Autodesk Inventor part; units mm, degrees
(part 2 of 2)
sketch "Sketch10" plane through (0, 6.35, 0) normal (0, 1, 0) x (1, 0, 0)
  line L0 (-0.1825, 29.2815) -> (-0.1825, 141.0415) projected
  arc A0 (-2.7225, 26.7415) -> (-0.1825, 29.2815) centre (-2.7225, 29.2815) ccw projected
  line L1 (-50.9825, 26.7415) -> (-2.7225, 26.7415) projected
  arc A1 (-53.5225, 29.2815) -> (-50.9825, 26.7415) centre (-50.9825, 29.2815) ccw projected
  line L2 (-53.5225, 141.0415) -> (-53.5225, 29.2815) projected
  arc A2 (-50.9825, 143.5815) -> (-53.5225, 141.0415) centre (-50.9825, 141.0415) ccw projected
  line L3 (-2.7225, 143.5815) -> (-50.9825, 143.5815) projected
  arc A3 (-0.1825, 141.0415) -> (-2.7225, 143.5815) centre (-2.7225, 141.0415) ccw projected
  line L4 (-2.405, 141.994) -> (-2.405, 141.359) projected
  line L5 (-3.04, 141.994) -> (-2.405, 141.994) projected
  line L6 (-3.04, 141.359) -> (-3.04, 141.994) projected
  line L7 (-2.405, 141.359) -> (-3.04, 141.359) projected
  line L8 (-50.665, 127.389) -> (-50.665, 126.754) projected
  line L9 (-51.3, 127.389) -> (-50.665, 127.389) projected
  line L10 (-51.3, 126.754) -> (-51.3, 127.389) projected
  line L11 (-50.665, 126.754) -> (-51.3, 126.754) projected
  line L12 (-50.665, 122.309) -> (-50.665, 121.674) projected
  line L13 (-51.3, 122.309) -> (-50.665, 122.309) projected
  line L14 (-51.3, 121.674) -> (-51.3, 122.309) projected
  line L15 (-50.665, 121.674) -> (-51.3, 121.674) projected
  line L16 (-50.665, 117.229) -> (-50.665, 116.594) projected
  line L17 (-51.3, 117.229) -> (-50.665, 117.229) projected
  line L18 (-51.3, 116.594) -> (-51.3, 117.229) projected
  line L19 (-50.665, 116.594) -> (-51.3, 116.594) projected
  line L20 (-50.665, 109.609) -> (-50.665, 108.974) projected
  line L21 (-51.3, 109.609) -> (-50.665, 109.609) projected
  line L22 (-51.3, 108.974) -> (-51.3, 109.609) projected
  line L23 (-50.665, 108.974) -> (-51.3, 108.974) projected
  line L24 (-50.665, 104.529) -> (-50.665, 103.894) projected
  line L25 (-51.3, 104.529) -> (-50.665, 104.529) projected
  line L26 (-51.3, 103.894) -> (-51.3, 104.529) projected
  line L27 (-50.665, 103.894) -> (-51.3, 103.894) projected
  line L28 (-50.665, 99.449) -> (-50.665, 98.814) projected
  line L29 (-51.3, 99.449) -> (-50.665, 99.449) projected
  line L30 (-51.3, 98.814) -> (-51.3, 99.449) projected
  line L31 (-50.665, 98.814) -> (-51.3, 98.814) projected
  line L32 (-2.405, 115.324) -> (-2.405, 114.689) projected
  line L33 (-3.04, 115.324) -> (-2.405, 115.324) projected
  line L34 (-3.04, 114.689) -> (-3.04, 115.324) projected
  line L35 (-2.405, 114.689) -> (-3.04, 114.689) projected
  line L36 (-3.04, 136.914) -> (-2.405, 136.914) projected
  line L37 (-3.04, 136.279) -> (-3.04, 136.914) projected
  line L38 (-2.405, 136.279) -> (-3.04, 136.279) projected
  line L39 (-2.405, 136.914) -> (-2.405, 136.279) projected
  line L40 (-3.04, 131.834) -> (-2.405, 131.834) projected
  line L41 (-3.04, 131.199) -> (-3.04, 131.834) projected
  line L42 (-2.405, 131.199) -> (-3.04, 131.199) projected
  line L43 (-2.405, 131.834) -> (-2.405, 131.199) projected
  line L44 (-3.04, 126.754) -> (-2.405, 126.754) projected
  line L45 (-3.04, 126.119) -> (-3.04, 126.754) projected
  line L46 (-2.405, 126.119) -> (-3.04, 126.119) projected
  line L47 (-2.405, 126.754) -> (-2.405, 126.119) projected
  line L48 (-3.04, 121.674) -> (-2.405, 121.674) projected
  line L49 (-3.04, 121.039) -> (-3.04, 121.674) projected
  line L50 (-2.405, 121.039) -> (-3.04, 121.039) projected
  line L51 (-2.405, 121.674) -> (-2.405, 121.039) projected
  line L52 (-2.405, 112.784) -> (-2.405, 112.149) projected
  line L53 (-3.04, 112.784) -> (-2.405, 112.784) projected
  line L54 (-3.04, 112.149) -> (-3.04, 112.784) projected
  line L55 (-2.405, 112.149) -> (-3.04, 112.149) projected
  line L56 (-2.405, 107.704) -> (-2.405, 107.069) projected
  line L57 (-3.04, 107.704) -> (-2.405, 107.704) projected
  line L58 (-3.04, 107.069) -> (-3.04, 107.704) projected
  line L59 (-2.405, 107.069) -> (-3.04, 107.069) projected
  line L60 (-2.405, 102.624) -> (-2.405, 101.989) projected
  line L61 (-3.04, 102.624) -> (-2.405, 102.624) projected
  line L62 (-3.04, 101.989) -> (-3.04, 102.624) projected
  line L63 (-2.405, 101.989) -> (-3.04, 101.989) projected
  line L64 (-2.405, 97.544) -> (-2.405, 96.909) projected
  line L65 (-3.04, 97.544) -> (-2.405, 97.544) projected
  line L66 (-3.04, 96.909) -> (-3.04, 97.544) projected
  line L67 (-2.405, 96.909) -> (-3.04, 96.909) projected
  circle A4 centre (-9.0725, 102.3065) radius 0.635 projected
  circle A5 centre (-9.0725, 104.8465) radius 0.635 projected
  circle A6 centre (-9.0725, 107.3865) radius 0.635 projected
  circle A7 centre (-9.0725, 109.9265) radius 0.635 projected
  circle A8 centre (-9.0725, 112.4665) radius 0.635 projected
  circle A9 centre (-9.0725, 115.0065) radius 0.635 projected
  circle A10 centre (-24.884, 29.9165) radius 0.3175 projected
  circle A11 centre (-26.535, 30.9325) radius 0.3175 projected
  circle A12 centre (-26.535, 32.9645) radius 0.3175 projected
  circle A13 centre (-23.36, 85.0345) radius 0.3175 projected
  circle A14 centre (-26.535, 86.0505) radius 0.3175 projected
  line L68 (-2.405, 100.084) -> (-2.405, 99.449) projected
  line L69 (-3.04, 100.084) -> (-2.405, 100.084) projected
  line L70 (-3.04, 99.449) -> (-3.04, 100.084) projected
  line L71 (-2.405, 99.449) -> (-3.04, 99.449) projected
  line L72 (-2.405, 105.164) -> (-2.405, 104.529) projected
  line L73 (-3.04, 105.164) -> (-2.405, 105.164) projected
  line L74 (-3.04, 104.529) -> (-3.04, 105.164) projected
  line L75 (-2.405, 104.529) -> (-3.04, 104.529) projected
  line L76 (-2.405, 110.244) -> (-2.405, 109.609) projected
  line L77 (-3.04, 110.244) -> (-2.405, 110.244) projected
  line L78 (-3.04, 109.609) -> (-3.04, 110.244) projected
  line L79 (-2.405, 109.609) -> (-3.04, 109.609) projected
  line L80 (-3.04, 119.134) -> (-2.405, 119.134) projected
  line L81 (-3.04, 118.499) -> (-3.04, 119.134) projected
  line L82 (-2.405, 118.499) -> (-3.04, 118.499) projected
  line L83 (-2.405, 119.134) -> (-2.405, 118.499) projected
  line L84 (-3.04, 124.214) -> (-2.405, 124.214) projected
  line L85 (-3.04, 123.579) -> (-3.04, 124.214) projected
  line L86 (-2.405, 123.579) -> (-3.04, 123.579) projected
  line L87 (-2.405, 124.214) -> (-2.405, 123.579) projected
  line L88 (-3.04, 129.294) -> (-2.405, 129.294) projected
  line L89 (-3.04, 128.659) -> (-3.04, 129.294) projected
  line L90 (-2.405, 128.659) -> (-3.04, 128.659) projected
  line L91 (-2.405, 129.294) -> (-2.405, 128.659) projected
  line L92 (-3.04, 134.374) -> (-2.405, 134.374) projected
  line L93 (-3.04, 133.739) -> (-3.04, 134.374) projected
  line L94 (-2.405, 133.739) -> (-3.04, 133.739) projected
  line L95 (-2.405, 134.374) -> (-2.405, 133.739) projected
  line L96 (-3.04, 139.454) -> (-2.405, 139.454) projected
  line L97 (-3.04, 138.819) -> (-3.04, 139.454) projected
  line L98 (-2.405, 138.819) -> (-3.04, 138.819) projected
  line L99 (-2.405, 139.454) -> (-2.405, 138.819) projected
  line L100 (-50.665, 96.909) -> (-50.665, 96.274) projected
  line L101 (-51.3, 96.909) -> (-50.665, 96.909) projected
  line L102 (-51.3, 96.274) -> (-51.3, 96.909) projected
  line L103 (-50.665, 96.274) -> (-51.3, 96.274) projected
  line L104 (-50.665, 101.989) -> (-50.665, 101.354) projected
  line L105 (-51.3, 101.989) -> (-50.665, 101.989) projected
  line L106 (-51.3, 101.354) -> (-51.3, 101.989) projected
  line L107 (-50.665, 101.354) -> (-51.3, 101.354) projected
  line L108 (-50.665, 107.069) -> (-50.665, 106.434) projected
  line L109 (-51.3, 107.069) -> (-50.665, 107.069) projected
  line L110 (-51.3, 106.434) -> (-51.3, 107.069) projected
  line L111 (-50.665, 106.434) -> (-51.3, 106.434) projected
  line L112 (-50.665, 114.689) -> (-50.665, 114.054) projected
  line L113 (-51.3, 114.689) -> (-50.665, 114.689) projected
  line L114 (-51.3, 114.054) -> (-51.3, 114.689) projected
  line L115 (-50.665, 114.054) -> (-51.3, 114.054) projected
  line L116 (-50.665, 119.769) -> (-50.665, 119.134) projected
  line L117 (-51.3, 119.769) -> (-50.665, 119.769) projected
  line L118 (-51.3, 119.134) -> (-51.3, 119.769) projected
  line L119 (-50.665, 119.134) -> (-51.3, 119.134) projected
  line L120 (-50.665, 124.849) -> (-50.665, 124.214) projected
  line L121 (-51.3, 124.849) -> (-50.665, 124.849) projected
  line L122 (-51.3, 124.214) -> (-51.3, 124.849) projected
  line L123 (-50.665, 124.214) -> (-51.3, 124.214) projected
  line L124 (-50.665, 129.929) -> (-50.665, 129.294) projected
  line L125 (-51.3, 129.929) -> (-50.665, 129.929) projected
  line L126 (-51.3, 129.294) -> (-51.3, 129.929) projected
  line L127 (-50.665, 129.294) -> (-51.3, 129.294) projected
  line L128 (-50.665, 132.469) -> (-50.665, 131.834) projected
  line L129 (-51.3, 132.469) -> (-50.665, 132.469) projected
  line L130 (-51.3, 131.834) -> (-51.3, 132.469) projected
  line L131 (-50.665, 131.834) -> (-51.3, 131.834) projected
  circle A15 centre (-47.1725, 96.5915) radius 0.635 projected
  circle A16 centre (-47.1725, 99.1315) radius 0.635 projected
  circle A17 centre (-47.1725, 101.6715) radius 0.635 projected
  circle A18 centre (-47.1725, 104.2115) radius 0.635 projected
  circle A19 centre (-47.1725, 106.7515) radius 0.635 projected
  circle A20 centre (-47.1725, 109.2915) radius 0.635 projected
  circle A21 centre (-47.1725, 114.3715) radius 0.635 projected
  circle A22 centre (-47.1725, 116.9115) radius 0.635 projected
  circle A23 centre (-47.1725, 119.4515) radius 0.635 projected
  circle A24 centre (-47.1725, 121.9915) radius 0.635 projected
  circle A25 centre (-47.1725, 124.5315) radius 0.635 projected
  circle A26 centre (-47.1725, 127.0715) radius 0.635 projected
  circle A27 centre (-47.1725, 129.6115) radius 0.635 projected
  circle A28 centre (-47.1725, 132.1515) radius 0.635 projected
  circle A29 centre (-6.5325, 97.2265) radius 0.635 projected
  circle A30 centre (-6.5325, 99.7665) radius 0.635 projected
  circle A31 centre (-6.5325, 102.3065) radius 0.635 projected
  circle A32 centre (-6.5325, 104.8465) radius 0.635 projected
  circle A33 centre (-6.5325, 107.3865) radius 0.635 projected
  circle A34 centre (-6.5325, 109.9265) radius 0.635 projected
  circle A35 centre (-6.5325, 112.4665) radius 0.635 projected
  circle A36 centre (-6.5325, 118.8165) radius 0.635 projected
  circle A37 centre (-6.5325, 121.3565) radius 0.635 projected
  circle A38 centre (-6.5325, 123.8965) radius 0.635 projected
  circle A39 centre (-6.5325, 126.4365) radius 0.635 projected
  circle A40 centre (-6.5325, 128.9765) radius 0.635 projected
  circle A41 centre (-6.5325, 131.5165) radius 0.635 projected
  circle A42 centre (-6.5325, 134.0565) radius 0.635 projected
  circle A43 centre (-6.5325, 136.5965) radius 0.635 projected
  circle A44 centre (-6.5325, 139.1365) radius 0.635 projected
  circle A45 centre (-6.5325, 115.0065) radius 0.635 projected
  circle A46 centre (-6.5325, 141.6765) radius 0.635 projected
  circle A47 centre (-10.3425, 141.6765) radius 0.635 projected
  circle A48 centre (-12.8825, 141.6765) radius 0.635 projected
  circle A49 centre (-15.4225, 141.6765) radius 0.635 projected
  circle A50 centre (-17.9625, 141.6765) radius 0.635 projected
  circle A51 centre (-20.5025, 141.6765) radius 0.635 projected
  circle A52 centre (-23.0425, 141.6765) radius 0.635 projected
  circle A53 centre (-25.5825, 141.6765) radius 0.635 projected
  circle A54 centre (-28.1225, 141.6765) radius 0.635 projected
  circle A55 centre (-30.6625, 141.6765) radius 0.635 projected
  circle A56 centre (-33.2025, 141.6765) radius 0.635 projected
  circle A57 centre (-35.7425, 141.6765) radius 0.635 projected
  circle A58 centre (-38.2825, 141.6765) radius 0.635 projected
  circle A59 centre (-40.8225, 141.6765) radius 0.635 projected
  circle A60 centre (-10.3425, 128.9765) radius 0.635 projected
  circle A61 centre (-10.3425, 131.5165) radius 0.635 projected
  circle A62 centre (-10.3425, 134.0565) radius 0.635 projected
  circle A63 centre (-10.3425, 136.5965) radius 0.635 projected
  circle A64 centre (-10.3425, 139.1365) radius 0.635 projected
  circle A65 centre (-12.8825, 128.9765) radius 0.635 projected
  circle A66 centre (-12.8825, 131.5165) radius 0.635 projected
  circle A67 centre (-12.8825, 134.0565) radius 0.635 projected
  circle A68 centre (-12.8825, 136.5965) radius 0.635 projected
  circle A69 centre (-12.8825, 139.1365) radius 0.635 projected
  circle A70 centre (-15.4225, 128.9765) radius 0.635 projected
  circle A71 centre (-15.4225, 131.5165) radius 0.635 projected
  circle A72 centre (-15.4225, 134.0565) radius 0.635 projected
  circle A73 centre (-15.4225, 136.5965) radius 0.635 projected
  circle A74 centre (-15.4225, 139.1365) radius 0.635 projected
  circle A75 centre (-17.9625, 128.9765) radius 0.635 projected
  circle A76 centre (-17.9625, 131.5165) radius 0.635 projected
  circle A77 centre (-17.9625, 134.0565) radius 0.635 projected
  circle A78 centre (-17.9625, 136.5965) radius 0.635 projected
  circle A79 centre (-17.9625, 139.1365) radius 0.635 projected
  circle A80 centre (-20.5025, 128.9765) radius 0.635 projected
  circle A81 centre (-20.5025, 131.5165) radius 0.635 projected
  circle A82 centre (-20.5025, 134.0565) radius 0.635 projected
  circle A83 centre (-20.5025, 136.5965) radius 0.635 projected
  circle A84 centre (-20.5025, 139.1365) radius 0.635 projected
  circle A85 centre (-23.0425, 128.9765) radius 0.635 projected
  circle A86 centre (-23.0425, 131.5165) radius 0.635 projected
  circle A87 centre (-23.0425, 134.0565) radius 0.635 projected
  circle A88 centre (-23.0425, 136.5965) radius 0.635 projected
  circle A89 centre (-23.0425, 139.1365) radius 0.635 projected
  circle A90 centre (-25.5825, 128.9765) radius 0.635 projected
  circle A91 centre (-25.5825, 131.5165) radius 0.635 projected
  circle A92 centre (-25.5825, 134.0565) radius 0.635 projected
  circle A93 centre (-25.5825, 136.5965) radius 0.635 projected
  circle A94 centre (-25.5825, 139.1365) radius 0.635 projected
  circle A95 centre (-28.1225, 128.9765) radius 0.635 projected
  circle A96 centre (-28.1225, 131.5165) radius 0.635 projected
  circle A97 centre (-28.1225, 134.0565) radius 0.635 projected
  circle A98 centre (-28.1225, 136.5965) radius 0.635 projected
  circle A99 centre (-28.1225, 139.1365) radius 0.635 projected
  circle A100 centre (-30.6625, 128.9765) radius 0.635 projected
  circle A101 centre (-30.6625, 131.5165) radius 0.635 projected
  circle A102 centre (-30.6625, 134.0565) radius 0.635 projected
  circle A103 centre (-30.6625, 136.5965) radius 0.635 projected
  circle A104 centre (-30.6625, 139.1365) radius 0.635 projected
  circle A105 centre (-33.2025, 128.9765) radius 0.635 projected
  circle A106 centre (-33.2025, 131.5165) radius 0.635 projected
  circle A107 centre (-33.2025, 134.0565) radius 0.635 projected
  circle A108 centre (-33.2025, 136.5965) radius 0.635 projected
  circle A109 centre (-33.2025, 139.1365) radius 0.635 projected
  circle A110 centre (-35.7425, 128.9765) radius 0.635 projected
  circle A111 centre (-35.7425, 131.5165) radius 0.635 projected
  circle A112 centre (-35.7425, 134.0565) radius 0.635 projected
  circle A113 centre (-35.7425, 136.5965) radius 0.635 projected
  circle A114 centre (-35.7425, 139.1365) radius 0.635 projected
  circle A115 centre (-38.2825, 128.9765) radius 0.635 projected
  circle A116 centre (-38.2825, 131.5165) radius 0.635 projected
  circle A117 centre (-38.2825, 134.0565) radius 0.635 projected
  circle A118 centre (-38.2825, 136.5965) radius 0.635 projected
  circle A119 centre (-38.2825, 139.1365) radius 0.635 projected
  circle A120 centre (-40.8225, 128.9765) radius 0.635 projected
  circle A121 centre (-40.8225, 131.5165) radius 0.635 projected
  circle A122 centre (-40.8225, 134.0565) radius 0.635 projected
  circle A123 centre (-40.8225, 136.5965) radius 0.635 projected
  circle A124 centre (-40.8225, 139.1365) radius 0.635 projected
  circle A125 centre (-43.3625, 128.9765) radius 0.635 projected
  circle A126 centre (-43.3625, 131.5165) radius 0.635 projected
  circle A127 centre (-43.3625, 134.0565) radius 0.635 projected
  circle A128 centre (-43.3625, 136.5965) radius 0.635 projected
  circle A129 centre (-43.3625, 139.1365) radius 0.635 projected
  circle A130 centre (-43.3625, 141.6765) radius 0.635 projected
  circle A131 centre (-50.9825, 29.2815) radius 1.5875 projected
  circle A132 centre (-50.9825, 91.5115) radius 1.5875 projected
  circle A133 centre (-2.7225, 91.5115) radius 1.5875 projected
  circle A134 centre (-2.7225, 29.2815) radius 1.5875 projected
  line L132 (-2.7225, 91.5115) -> (-50.9825, 91.5115)
  point P0 (0, 0)
  constraints: 2 end point, 1 horizontal
equation "\"d1\" = BaseWidth"
equation "\"d2\" = WallConA"
equation "\"d3\" = WallConB"
equation "\"d5\" = d2"
equation "\"d6\" = WallConSpace"
equation "\"d7\" = d4"
equation "\"d8\" = d2"
equation "\"d9\" = d6"
equation "\"d10\" = d4"
equation "\"d11\" = -0.8 * d13 + 0.2 * d12"
equation "\"d13\" = 0.111111 * d12"
equation "\"d14\" = WallConA"
equation "\"d15\" = d14"
equation "\"d16\" = d13"
equation "\"d17\" = d15"
equation "\"d18\" = d20"
equation "\"d22\" = d17"
equation "\"d23\" = d25"
equation "\"d27\" = d11"
equation "\"d28\" = d27"
equation "\"d29\" = d11"
equation "\"d34\" = d36"
equation "\"d35\" = d37"
equation "\"d40\" = d7"
equation "\"d41\" = d5"
equation "\"d42\" = d5"
equation "\"d43\" = d41"
equation "\"d44\" = d42"
equation "\"d45\" = d41"
equation "\"d46\" = d42"
equation "\"d47\" = d41"
equation "\"d48\" = d42"
equation "\"d50\" = 0.5 * d49"
equation "\"d52\" = d51"
equation "\"d56\" = d54"
equation "\"d57\" = 0.5 * d55"
equation "\"d4\" = WallConSpace"
equation "\"d20\" = 0.111111 * d21"
equation "\"d25\" = 0.111111 * d26"
equation "\"d36\" = d38"
equation "\"d37\" = d39"
equation "\"BaseWidth\" = 166.624"
equation "\"WallConA\" = 8.89"
equation "\"WallConB\" = 23.803429"
equation "\"WallConSpace\" = 23.803429"
equation "\"d21\" = 127"
equation "\"d26\" = 127"
equation "\"d38\" = 8.89"
equation "\"d39\" = 16.546286"
body "Solid1"
